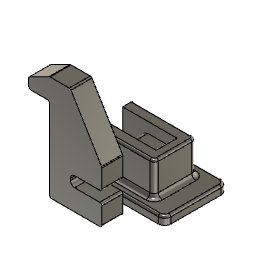
ac_filler_support (Autodesk Fusion 360 design; units mm, degrees)
Autodesk Fusion 360 part; units mm, degrees
sketch "Sketch1" plane through (0, 0, 0) normal (0, 1, 0) x (1, 0, 0)
  line L0 (25, 0) -> (15, 0)
  line L1 (15, 0) -> (15, -40)
  line L2 (25, -15) -> (25, -10)
  line L3 (15, -40) -> (5, -40)
  line L4 (5, -40) -> (5, -45)
  line L5 (15, -50) -> (25, -50)
  line L6 (5, -45) -> (15, -50)
  line L7 (25, 0) -> (40, 0)
  line L8 (40, 0) -> (40, -10)
  line L9 (40, -10) -> (25, -10)
  line L10 (25, -15) -> (40, -15)
  line L11 (40, -15) -> (40, -25)
  line L12 (40, -25) -> (25, -50)
  constraint horizontal L0
  constraint vertical L1
  constraint vertical L2
  constraint horizontal L3
  constraint vertical L4
  constraint horizontal L5
  constraint horizontal L7
  constraint vertical L8
  constraint horizontal L9
  constraint perpendicular L2 L10
  constraint perpendicular L10 L11
extrude "Extrude1" add sketch "Sketch1" along normal blind 10 makes body 1
fillet "Fillet1" radius 1 10 edges at (15, 5, 50) (25, 5, 50) (40, 5, 25) (5, 5, 45) (5, 5, 40) (15, 5, 40) (15, 5, 0) (40, 5, 0) (40, 5, 10) (40, 5, 15) on bodies 1
fillet "Fillet2" radius 2 2 edges at (25, 5, 15) (25, 5, 10) on bodies 1
sketch "Sketch2" plane through (0, 0, 0) normal (0, 0, 1) x (1, 0, 0)
  line L0 (25, 15) -> (55, 15)
  line L1 (55, 15) -> (55, 45)
  line L2 (55, 45) -> (25, 45)
  line L3 (25, 35) -> (40, 35)
  line L4 (40, 35) -> (40, 25)
  line L5 (40, 25) -> (25, 25)
  line L6 (25, 45) -> (25, 35)
  line L7 (25, 25) -> (25, 15)
  constraint horizontal L0
  constraint vertical L1
  constraint horizontal L2
  constraint vertical L6
  constraint horizontal L3
  constraint vertical L4
  constraint horizontal L5
  constraint collinear L6 L7
extrude "Extrude2" add sketch "Sketch2" along normal blind 4 separate body makes body 2
sketch "Sketch3" plane through (0, 0, 4) normal (0, 0, 1) x (-1, 0, 0)
  line L0 (-25, -25) -> (-25, -15)
  line L1 (-25, -15) -> (-55, -15)
  line L2 (-55, -15) -> (-55, -45)
  line L3 (-55, -45) -> (-25, -45)
  line L4 (-25, -45) -> (-25, -35)
  line L5 (-25, -35) -> (-40, -35)
  line L6 (-40, -35) -> (-40, -25)
  line L7 (-40, -25) -> (-25, -25)
  line L8 (-25, -35) -> (-40, -35)
  line L9 (-40, -25) -> (-25, -25)
  line L10 (-25, -20) -> (-45, -20)
  line L11 (-45, -20) -> (-45, -40)
  line L12 (-45, -40) -> (-25, -40)
  constraint coincident L4.end L5.start
  constraint coincident L5.end L6.start
  constraint coincident L6.end L7.start
  constraint coincident L0.start L7.end
  constraint midpoint L0 L10.start
  constraint perpendicular L0 L10
  constraint perpendicular L10 L11
  constraint midpoint L4 L12.end
  constraint perpendicular L4 L12
extrude "Extrude3" add sketch "Sketch3" along normal blind 6 contours L0 L4 L5 L6 L7 L8 L9 L10 L11 L12 bodies 2
sketch "Sketch4" plane through (0, 0, 10) normal (0, 0, 1) x (-1, 0, 0)
  line L0 (-45, -40) -> (-25, -40)
  line L1 (-25, -40) -> (-25, -35)
  line L2 (-25, -35) -> (-40, -35)
  line L3 (-40, -35) -> (-40, -25)
  line L4 (-40, -25) -> (-25, -25)
  line L5 (-25, -25) -> (-25, -20)
  line L6 (-25, -20) -> (-45, -20)
  line L7 (-45, -20) -> (-45, -40)
  line L8 (-25, -40) -> (-45, -40)
  line L9 (-45, -40) -> (-45, -20)
  line L10 (-45, -20) -> (-25, -20)
  line L11 (-25, -20) -> (-25, -40)
  constraint horizontal L8
  constraint vertical L9
  constraint horizontal L10
  constraint vertical L11
  constraint coincident L6.end L7.start
  constraint coincident L0.end L1.start
extrude "Extrude4" add sketch "Sketch4" along normal blind 5 bodies 2
sketch "Sketch5" plane through (0, 0, 15) normal (0, 0, 1) x (-1, 0, 0)
  line L0 (-25, -20) -> (-45, -20)
  line L1 (-45, -20) -> (-45, -40)
  line L2 (-45, -40) -> (-25, -40)
  line L3 (-25, -40) -> (-25, -20)
  line L4 (-25, -40) -> (-45, -40)
  line L5 (-45, -20) -> (-25, -20)
  line L6 (-25, -25) -> (-40, -25)
  line L7 (-40, -25) -> (-40, -35)
  line L8 (-40, -35) -> (-25, -35)
  constraint coincident L2.end L3.start
  constraint coincident L1.end L2.start
  constraint coincident L0.end L1.start
  constraint coincident L0.start L3.end
  constraint coincident L3 L6.start
  constraint perpendicular L3 L6
  constraint perpendicular L6 L7
  constraint coincident L3 L8.end
  constraint perpendicular L3 L8
extrude "Extrude5" add sketch "Sketch5" along normal blind 5 contours L0 L1 L2 L3 L4 L5 L6 L7 L8 bodies 2
fillet "Fillet3" radius 3 1 edges at (55, 15, 2) on bodies 2
fillet "Fillet4" radius 3 1 edges at (55, 45, 2) on bodies 2
fillet "Fillet5" radius 2 2 edges at (25, 30, 15) (25, 30, 10) on bodies 2
sketch "Sketch6" plane through (25, 0, 0) normal (-1, 0, 0) x (0, -1, 0)
  line L0 (-35, 0) -> (-35, 12)
  line L1 (-35, 12) -> (-25, 12)
  line L2 (-25, 12) -> (-25, 0)
  line L3 (-25, 0) -> (-15, 0)
  line L4 (-15, 0) -> (-15, 4)
  line L5 (-15, 4) -> (-20, 4)
  line L6 (-20, 4) -> (-20, 20)
  line L7 (-20, 20) -> (-25, 20)
  line L8 (-25, 20) -> (-25, 13)
  line L9 (-25, 13) -> (-35, 13)
  line L10 (-35, 13) -> (-35, 20)
  line L11 (-35, 20) -> (-40, 20)
  line L12 (-40, 20) -> (-40, 4)
  line L13 (-40, 4) -> (-45, 4)
  line L14 (-45, 4) -> (-45, 0)
  line L15 (-45, 0) -> (-35, 0)
  line L16 (-40, 4) -> (-45, 4)
  line L17 (-45, 0) -> (-35, 0)
  line L18 (-35, 20) -> (-40, 20)
  line L19 (-25, 20) -> (-25, 0)
  line L20 (-15, 0) -> (-15, 4)
  line L21 (-20, 4) -> (-20, 20)
  line L22 (-35, 20) -> (-35, 0)
  constraint coincident L12.end L13.start
  constraint coincident L13.end L14.start
  constraint coincident L14.end L15.start
  constraint coincident L0.start L15.end
  constraint coincident L10.end L11.start
  constraint coincident L11.end L12.start
  constraint coincident L7.end L8.start
  constraint coincident L2.end L3.start
  constraint coincident L3.end L4.start
  constraint coincident L4.end L5.start
  constraint coincident L5.end L6.start
  constraint coincident L6.end L7.start
extrude "Extrude6" add sketch "Sketch6" along normal blind 10 contours L0 L10 L11 L12 L13 L14 L15 L16 L17 L18 L22 | L2 L3 L4 L5 L6 L7 L8 L19 L20 L21 bodies 2
fillet "Fillet6" radius 1 5 edges at (40, 30, 15) (40, 30, 20) (45, 30, 20) (30, 40, 20) (30, 20, 20) on bodies 2
fillet "Fillet7" radius 1 1 edges at (40, 30, 10) on bodies 2
fillet "Fillet8" radius 2 4 edges at (45, 20, 11.5) (44.7071, 20.2929, 19.7071) (45, 40, 11.5) (44.7071, 39.7071, 19.7071) on bodies 2
fillet "Fillet9" radius 1 5 edges at (33.5, 45, 4) (54.1213, 44.1213, 4) (55, 30, 4) (54.1213, 15.8787, 4) (33.5, 15, 4) on bodies 2
fillet "Fillet10" radius 2 5 edges at (29, 40, 4) (44.4142, 39.4142, 4) (45, 30, 4) (44.4142, 20.5858, 4) (29, 20, 4) on bodies 2
